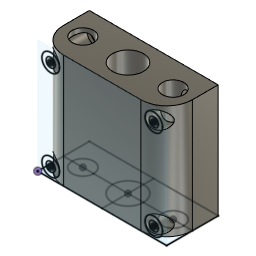
Z-Holder (Autodesk Fusion 360 design; units mm, degrees)
Autodesk Fusion 360 part; units mm, degrees
note: some values were not read from the file. Set by a fixed rule: which sketch regions a step uses.
sketch "Skizze1" plane through (0, 0, 0) normal (0, 0, 1) x (1, 0, 0)
  line L0 (0, 0) -> (50, 0)
  line L1 (50, 0) -> (50, 20)
  line L2 (50, 20) -> (0, 20)
  line L3 (0, 20) -> (0, 0)
  line L4 (0, 10) -> (50, 10)
  circle A0 centre (7.5, 10) radius 4.15
  circle A1 centre (42.5, 10) radius 4.15
  line L5 (25, 20) -> (25, 0)
  circle A2 centre (25, 10) radius 6
  dimension "d1" = 50
  dimension "d2" = 20
  dimension "d3" = 8.3
  dimension "d4" = 8.3
  dimension "d5" = 17.5
  dimension "d6" = 17.5
  dimension "d7" = 12
  constraint horizontal L0
  constraint vertical L1
  constraint horizontal L2
  constraint vertical L3
  constraint coincident L0.start L3.end
  constraint midpoint L3 L4.start
  constraint midpoint L1 L4.end
  constraint coincident L4 A0.centre
  constraint coincident L4 A1.centre
  constraint midpoint L2 L5.start
  constraint midpoint L0 L5.end
  constraint midpoint L4 A2.centre
  measures "d1" distance of L0.start L0.end
  measures "d2" distance of L0.start L2.end
  measures "d3" diameter of A0
  measures "d4" diameter of A1
  measures "d5" distance of A0.centre L5
  measures "d6" distance of A1.centre L5
  measures "d7" diameter of A2
extrude "Extrusion1" add sketch "Skizze1" along normal blind 44 contours L0 L3 L4 A0 L5 A2 | L0 L1 L4 A1 L5 A2 | L2 L3 L4 A0 L5 A2 | L1 L2 L4 A1 L5 A2
extrude "Extrusion4" add sketch "Skizze1" along normal blind 19 contours L4 A0 | L4 A0 | L4 A1 | L4 A1
sketch "Skizze2" plane through (0, 0, 0) normal (0, -1, 0) x (1, 0, 0)
  line L0 (0, 0) -> (50, 0)
  line L1 (50, 0) -> (50, 44)
  line L2 (50, 44) -> (0, 44)
  line L3 (0, 44) -> (0, 0)
  circle A0 centre (5, 39) radius 1.75
  circle A1 centre (45, 39) radius 1.75
  circle A2 centre (45, 39) radius 3.4
  circle A3 centre (5, 39) radius 3.4
  circle A4 centre (5, 4) radius 1.75
  circle A5 centre (5, 4) radius 3.4
  circle A6 centre (45, 4) radius 1.75
  circle A7 centre (45, 4) radius 3.4
  dimension "d10" = 5
  dimension "d11" = 5
  dimension "d12" = 5
  dimension "d13" = 5
  dimension "d14" = 3.5
  dimension "d15" = 3.5
  dimension "d16" = 6.8
  dimension "d23" = 40
  dimension "d24" = 40
  dimension "d25" = 5
  dimension "d26" = 5
  constraint concentric A1 A2
  constraint concentric A0 A3
  constraint equal A2 A3
  constraint concentric A4 A5
  constraint concentric A6 A7
  constraint equal A3 A5
  constraint equal A3 A7
  constraint equal A0 A4
  constraint equal A4 A6
  measures "d10" distance of L2 A0.centre
  measures "d11" distance of L3 A0.centre
  measures "d12" distance of L1 A1.centre
  measures "d13" distance of L2 A1.centre
  measures "d14" diameter of A0
  measures "d15" diameter of A1
  measures "d16" diameter of A2
  measures "d23" distance of L2 A4.centre
  measures "d24" distance of L2 A6.centre
  measures "d25" distance of L3 A4.centre
  measures "d26" distance of L1 A6.centre
extrude "Extrusion2" cut sketch "Skizze2" against normal blind 20 contours A0 | A1 | A4 | A6
extrude "Extrusion3" cut sketch "Skizze2" against normal blind 17.5 contours A2 | A3 | A5 | A7
fillet "Abrundung1" radius 10 2 edges at (50, 0, 22) (0, 0, 22)
